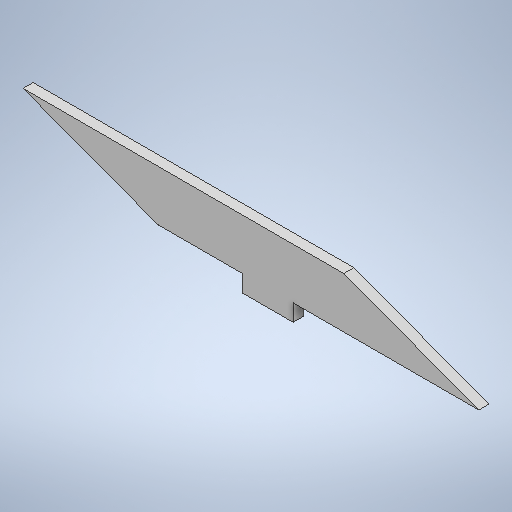
# Autodesk Inventor part: Hinge Siderail 2
Saved by Autodesk Inventor 2025.1 (Build 291241020, 241B)
## iProperties
Created: 2024-10-28
Part Number: Hinge Siderail 2
Material: Generic
Document SubType Name: Modeling
Designer: aly_g
Density: 1 g/cm^3
Appearance: Default
Author: aly_g
Autodesk Inventor part; units mm, degrees
ref_plane "YZ Plane" through (0, 0, 0) normal (1, 0, 0) x (0, 1, 0)
ref_plane "XZ Plane" through (0, 0, 0) normal (0, 1, 0) x (-1, 0, 0)
ref_plane "XY Plane" through (0, 0, 0) normal (0, 0, 1) x (1, 0, 0)
sketch "Sketch1" plane through (0, 0, 0) normal (0, 0, 1) x (1, 0, 0)
  line L0 (0, 0) -> (95, 0)
  line L1 (25, 0) -> (40, 0)
  line L2 (40, 0) -> (40, -5)
  line L3 (40, -5) -> (25, -5)
  line L4 (25, -5) -> (25, 0)
  line L5 (0, 0) -> (-40, 15)
  line L6 (-40, 15) -> (55, 15)
  line L7 (55, 15) -> (95, 0)
  dimension "d0" = 95
  dimension "d6" = 15
  dimension "d7" = 5
  dimension "d8" = 25
  dimension "d21" = 15
  dimension "d22" = 40
  constraints: 16 end point, 4 parallel, 2 horizontal, 1 perpendicular, 1 point on line
  measures "d0" distance of L0.start L0.end
  measures "d6" distance of L2.end L3.end
  measures "d7" distance of L1.end L2.end
  measures "d8" distance of L0.start L1.start
  measures "d21" vertical distance of L6.end L0.end
  measures "d22" horizontal distance of L6.end L0.end
extrude "Extrusion1" add sketch "Sketch1" along normal blind 3
body "Solid1"
